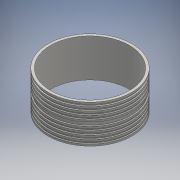
# Autodesk Inventor part: Wheel_covering_ENES100OSV-spencermical-3-30-pm 3-5-16-saturday
Saved by Autodesk Inventor 2016 (Build 200138000, 138)
## iProperties
Created: 2016-03-05
Part Number: Wheel_covering_ENES100OSV-spencermical-3-30-pm 3-5-16-saturday
Material: Generic
Document SubType Name: Modeling
Designer: Spencer
Density: 1 g/cm^3
Appearance: Default
Author: Spencer
Autodesk Inventor part; units mm, degrees
ref_plane "YZ Plane" through (0, 0, 0) normal (1, 0, 0) x (0, 1, 0)
ref_plane "XZ Plane" through (0, 0, 0) normal (0, 1, 0) x (-1, 0, 0)
ref_plane "XY Plane" through (0, 0, 0) normal (0, 0, 1) x (1, 0, 0)
sketch "Sketch1" plane through (0, 0, 0) normal (1, 0, 0) x (0, 1, 0)
  line L0 (0, 0) -> (61.5, 0) construction
  line L1 (61.5, 0) -> (61.9, 0) construction
  line L2 (61.9, 0) -> (61.9, -30)
  line L3 (61.9, 0) -> (61.9, 30)
  line L4 (61.9, 30) -> (65.9, 30)
  line L5 (65.9, -30) -> (61.9, -30)
  line L6 (61.9, -30) -> (61.9, 30)
  line L7 (65.9, 27) -> (63.9, 27)
  line L8 (63.9, 27) -> (63.9, 24)
  line L9 (63.9, 24) -> (65.9, 24)
  line L10 (65.9, 21) -> (63.9, 21)
  line L11 (63.9, 21) -> (63.9, 18)
  line L12 (63.9, 18) -> (65.9, 18)
  line L13 (65.9, 15) -> (63.9, 15)
  line L14 (63.9, 15) -> (63.9, 12)
  line L15 (63.9, 12) -> (65.9, 12)
  line L16 (65.9, 9) -> (63.9, 9)
  line L17 (63.9, 9) -> (63.9, 6)
  line L18 (63.9, 6) -> (65.9, 6)
  line L19 (65.9, 30) -> (65.9, 27)
  line L20 (65.9, 24) -> (65.9, 21)
  line L21 (65.9, 18) -> (65.9, 15)
  line L22 (65.9, 12) -> (65.9, 9)
  line L23 (65.9, 3) -> (63.9, 3)
  line L24 (63.9, 3) -> (63.9, 0)
  line L25 (63.9, 0) -> (65.9, 0)
  line L26 (65.9, 0) -> (61.9, 0) construction
  line L27 (65.9, 0) -> (61.9, 0) construction
  line L28 (65.9, 6) -> (65.9, 3)
  line L29 (65.9, -27) -> (63.9, -27)
  line L30 (63.9, -27) -> (63.9, -24)
  line L31 (63.9, -24) -> (65.9, -24)
  line L32 (65.9, -21) -> (63.9, -21)
  line L33 (63.9, -21) -> (63.9, -18)
  line L34 (63.9, -18) -> (65.9, -18)
  line L35 (65.9, -15) -> (63.9, -15)
  line L36 (63.9, -15) -> (63.9, -12)
  line L37 (63.9, -12) -> (65.9, -12)
  line L38 (65.9, -9) -> (63.9, -9)
  line L39 (63.9, -9) -> (63.9, -6)
  line L40 (63.9, -6) -> (65.9, -6)
  line L41 (65.9, -30) -> (65.9, -27)
  line L42 (65.9, -24) -> (65.9, -21)
  line L43 (65.9, -18) -> (65.9, -15)
  line L44 (65.9, -12) -> (65.9, -9)
  line L45 (65.9, -3) -> (63.9, -3)
  line L46 (63.9, -3) -> (63.9, 0)
  line L47 (65.9, -6) -> (65.9, -3)
  line L48 (65.9, -3) -> (65.9, -12)
  line L49 (65.9, -15) -> (65.9, -30)
  line L50 (0, -42) -> (0, 42) projected
  dimension "d0" = 61.5
  dimension "d1" = 0.4
  dimension "d2" = 30
  dimension "d3" = 4
  dimension "d4" = 3
  dimension "d5" = 3
  dimension "d6" = 3
  dimension "d7" = 3
  dimension "d8" = 3
  dimension "d9" = 3
  dimension "d10" = 3
  dimension "d11" = 3
  constraints: 100 end point, 19 symmetric about line, 13 parallel, 12 perpendicular, 8 horizontal, 4 point on line, 3 collinear, 1 vertical
  measures "d0" distance of L0.start L0.end
  measures "d1" distance of L0.end L1.end
  measures "d2" distance of L1.end L2.end
  measures "d3" distance of L5.start L5.end
  measures "d4" distance from line of L7.end L4
  measures "d5" distance of L7.end L8.end
  measures "d6" distance of L10.end L11.end
  measures "d7" distance between parallel lines of L10 L9
  measures "d8" distance between parallel lines of L13 L12
  measures "d9" distance between parallel lines of L16 L15
  measures "d10" distance between parallel lines of L23 L18
  measures "d11" distance of L23.end L24.end
revolve "Revolution1" add sketch "Sketch1" angle 360 about axis through (0, 0, -10) along (0, 0, 1) contours L3 L4 L19 L7 L8 L9 L20 L10 L11 L12 L21 L13 L14 L15 L22 L16 L17 L18 L28 L23 L24 L46 L45 L47 L40 L39 L38 L44 L37 L36 L35 L43 L34 L33 L32 L42 L31 L30 L29 L41 L5 L2
body "Solid1"
